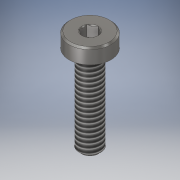
# Autodesk Inventor part: 48-0280
Saved by Autodesk Inventor 2018 (Build 220112000, 112)
## iProperties
Manager: Bradley
Company: Zetta & Zepto Technology
Created: 2016-07-03
Part Number: 48-0280
Material: Stainless Steel
Document SubType Name: Modeling
Designer: Bradley
Density: 8 g/cm^3
Appearance: Semi-Polished
Description: SCM4006-3H3
Stock Number: 80110
Author: Bradley
Autodesk Inventor part; units mm, degrees
ref_plane "YZ Plane" through (0, 0, 0) normal (1, 0, 0) x (0, 1, 0)
ref_plane "XZ Plane" through (0, 0, 0) normal (0, 1, 0) x (-1, 0, 0)
ref_plane "XY Plane" through (0, 0, 0) normal (0, 0, 1) x (1, 0, 0)
sketch "Sketch1" plane through (0, 0, 0) normal (0, 0, 1) x (1, 0, 0)
  line L0 (0, 4.675) -> (0, -4.675)
  line L1 (0, -4.675) -> (0.75, -4.675)
  line L2 (0.75, -4.675) -> (1, -4.425)
  line L3 (1, -4.425) -> (1, 3.225)
  line L4 (1.1, 3.325) -> (1.9, 3.325)
  line L5 (1.9, 3.325) -> (1.9, 4.525)
  line L6 (1.75, 4.675) -> (0, 4.675)
  arc A0 (1.1, 3.325) -> (1, 3.225) centre (1.1, 3.225) ccw
  line L7 (1.75, 4.675) -> (1.9, 4.525)
  point P0 (0, 0)
  point P1 (1.9, 4.675)
  point P2 (0, 0)
  dimension "d0" = 3.8
  dimension "d1" = 1.35
  dimension "d3" = 2
  dimension "d4" = 2.2
  dimension "d5" = 135
  dimension "d6" = 0.25
  dimension "d7" = 8
  dimension "d18" = 0.15
  dimension "d22" = 0.15
  constraints: 18 end point, 4 perpendicular, 4 point on line, 2 point on circle, 2 tangent, 1 centre point, 1 coincident, 1 midpoint, 1 parallel, 1 vertical
  measures "d0" diameter of L5 L0
  measures "d1" distance of L4.end point (1.9, 4.675)
  measures "d3" diameter of L3 L0
  measures "d4" diameter of L4.start L0
  measures "d5" angle of L3 L2
  measures "d6" horizontal distance of L1.end L2.end
  measures "d7" distance between parallel lines of L1 L4
  measures "d18" distance of L6.start point (1.9, 4.675)
  measures "d22" horizontal distance of L6.start L5.end
revolve "Revolution1" add sketch "Sketch1" angle 360 about axis through (0, 4.675, 0) along (0, -1, 0)
sketch "Sketch2" plane through (0, 4.675, 0) normal (0, 1, 0) x (1, 0, 0)
  line L0 (0, -0.7506) -> (-0.65, -0.3753)
  line L1 (-0.65, -0.3753) -> (-0.65, 0.3753)
  line L2 (-0.65, 0.3753) -> (0, 0.7506)
  line L3 (0, 0.7506) -> (0.65, 0.3753)
  line L4 (0.65, 0.3753) -> (0.65, -0.3753)
  line L5 (0.65, -0.3753) -> (0, -0.7506)
  point P0 (0, 0)
  point P1 (0, 0)
  dimension "d11" = 1.3
  constraints: 12 end point, 1 coincident, 1 vertical, 13 other
  measures "d11" distance between parallel lines of L4 L1
extrude "Extrusion1" cut sketch "Sketch2" against normal blind 1
thread "Thread1" size "M2x0.4" class "6g" standard "ANSI Metric M Profile" full length
sketch "Sketch3" plane through (0, 0, 0) normal (1, 0, 0) x (0, 1, 0)
  line L0 (4.675, 0.7506) -> (4.675, 0.3753) projected
  line L1 (4.675, 0.7506) -> (4.175, 0.2506)
  line L2 (4.175, 0.2506) -> (4.675, 0.2506)
  line L3 (4.675, 0.2506) -> (4.675, 0.7506)
  line L4 (-0.7, 0) -> (4.2, 0) projected
  point P0 (0, 0)
  dimension "d16" = 0.5
  constraints: 6 end point, 3 perpendicular
  measures "d16" distance of L2.end L0.start
revolve "Revolution2" cut sketch "Sketch3" angle 360 about axis through (0, -10, 0) along (0, 1, 0)
equation "\"d22\" = d18"
body "Solid1"
